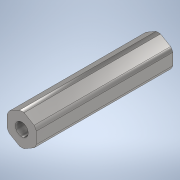
# Autodesk Inventor part: PulleyShaft
Saved by Autodesk Inventor 2020 (Build 240168000, 168)
## iProperties
Created: 2019-06-24
Part Number: PulleyShaft
Material: Steel, Carbon
Document SubType Name: Modeling
Designer: Connor
Density: 7.85 g/cm^3
Appearance: Semi-Polished
Author: Connor
Autodesk Inventor part; units mm, degrees
ref_plane "YZ Plane" through (0, 0, 0) normal (1, 0, 0) x (0, 1, 0)
ref_plane "XZ Plane" through (0, 0, 0) normal (0, 1, 0) x (-1, 0, 0)
ref_plane "XY Plane" through (0, 0, 0) normal (0, 0, 1) x (1, 0, 0)
sketch "Sketch1" plane through (0, 0, 0) normal (0, 0, 1) x (1, 0, 0)
  line L0 (0, 5.4993) -> (4.7625, 2.7496)
  line L1 (4.7625, 2.7496) -> (4.7625, -2.7496)
  line L2 (4.7625, -2.7496) -> (0, -5.4993)
  line L3 (0, -5.4993) -> (-4.7625, -2.7496)
  line L4 (-4.7625, -2.7496) -> (-4.7625, 2.7496)
  line L5 (-4.7625, 2.7496) -> (0, 5.4993)
  circle A0 centre (0, 0) radius 5.125
  circle A1 centre (0, 0) radius 2.0955
  point P0 (-4.0208, 3.1778)
  point P1 (-4.7625, 1.8932)
  point P2 (-4.7625, -1.8932)
  point P3 (-4.0208, -3.1778)
  point P4 (-0.7417, -5.071)
  point P5 (0.7417, -5.071)
  point P6 (4.0208, -3.1778)
  point P7 (4.7625, -1.8932)
  point P8 (4.7625, 1.8932)
  point P9 (4.0208, 3.1778)
  point P10 (0.7417, 5.071)
  point P11 (-0.7417, 5.071)
  dimension "d0" = 9.525
  dimension "d6" = 10.25
  dimension "d7" = 4.191
  constraints: 12 end point, 3 coincident, 2 centre point, 1 vertical alignment, 13 other
  measures "d0" distance between parallel lines of L1 L4
  measures "d6" diameter of A0
  measures "d7" diameter of A1
extrude "Extrusion1" add sketch "Sketch1" along normal mid plane 44.45 contours L0 A0 L1 L2 L3 L4 L5
body "Solid1"
